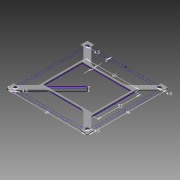
# Autodesk Inventor part: BattHolder
Saved by Autodesk Inventor 2014 SP1 (Build 180222100, 222)
## iProperties
Created: 2015-03-30
Part Number: BattHolder
Material: Generic
Document SubType Name: Modeling
Designer: Erin
Density: 1 g/cm^3
Appearance: Default
Author: Erin
Autodesk Inventor part; units mm, degrees
note: some values were not read from the file. Chosen so that the rebuilt part matches the saved one: sketch regions of "Extrusion2".
ref_plane "YZ Plane" through (0, 0, 0) normal (1, 0, 0) x (0, 1, 0)
ref_plane "XZ Plane" through (0, 0, 0) normal (0, 1, 0) x (-1, 0, 0)
ref_plane "XY Plane" through (0, 0, 0) normal (0, 0, 1) x (1, 0, 0)
sketch "Sketch1" plane through (0, 0, 0) normal (0, 0, 1) x (1, 0, 0)
  line L0 (-48, 48) -> (48, 48) construction
  line L1 (48, 48) -> (48, -48) construction
  line L2 (48, -48) -> (-48, -48) construction
  line L3 (-48, -48) -> (-48, 48) construction
  circle A0 centre (-45, 45) radius 2.25
  circle A1 centre (45, 45) radius 2.25
  line L4 (45, 45) -> (-45, 45) construction
  line L5 (-45, 45) -> (-45, -45) construction
  line L6 (-45, -45) -> (45, -45) construction
  line L7 (45, -45) -> (45, 45) construction
  circle A2 centre (45, -45) radius 2.25
  circle A3 centre (-45, -45) radius 2.25
  line L8 (-50.5, -50.5) -> (-42, -50.5)
  line L9 (-42, -50.5) -> (-42, -42)
  line L10 (-42, -42) -> (-50.5, -42)
  line L11 (-50.5, -42) -> (-50.5, -50.5)
  line L12 (0, 0) -> (-48, -48) construction
  line L13 (-33, 26.5) -> (33, 26.5)
  line L14 (33, 26.5) -> (33, -26.5)
  line L15 (33, -26.5) -> (-33, -26.5)
  line L16 (-33, -26.5) -> (-33, 26.5)
  line L17 (-2.4749, 2.4749) -> (2.4749, -2.4749)
  line L18 (2.4749, -2.4749) -> (-42.5251, -47.4749)
  line L19 (-42.5251, -47.4749) -> (-47.4749, -42.5251)
  line L20 (-47.4749, -42.5251) -> (-2.4749, 2.4749)
  line L21 (0, 0) -> (-45, -45) construction
  line L22 (31, 24.5) -> (-31, 24.5)
  line L23 (-31, 24.5) -> (-31, -24.5)
  line L24 (-31, -24.5) -> (31, -24.5)
  line L25 (31, -24.5) -> (31, 24.5)
  point P0 (0, 48)
  point P1 (48, 0)
  point P2 (33, 0)
  point P3 (0, 26.5)
  dimension "d0" = 96
  dimension "d1" = 96
  dimension "d2" = 4.5
  dimension "d3" = 4.5
  dimension "d4" = 3
  dimension "d5" = 4.5
  dimension "d6" = 4.5
  dimension "d9" = 3
  dimension "d10" = 3
  dimension "d11" = 66
  dimension "d12" = 53
  dimension "d13" = 7
  dimension "d14" = 0
  dimension "d23" = 5.5
  dimension "d24" = 5.5
  dimension "d25" = 2
  constraints: 52 end point, 12 parallel, 6 midpoint, 6 perpendicular, 4 centre point, 4 coincident, 3 horizontal, 2 horizontal alignment, 2 vertical alignment, 1 collinear, 6 other
  measures "d0" distance of L1.end L2.end
  measures "d1" distance of L0.end L1.end
  measures "d2" diameter of A0
  measures "d3" diameter of A1
  measures "d4" distance between parallel lines of L4 L0
  measures "d5" diameter of A2
  measures "d6" diameter of A3
  measures "d9" distance from line of A3.centre L10
  measures "d10" distance from line of A3.centre L9
  measures "d11" distance of L13.start L13.end
  measures "d12" distance of L13.end L14.end
  measures "d13" distance of L17.start L17.end
  measures "d14" distance from line of L5.end L19
  measures "d23" distance from line of L11 A3.centre
  measures "d24" distance from line of A3.centre L8
  measures "d25" distance between parallel lines of L22 L13
extrude "Extrusion1" add sketch "Sketch1" along normal blind 1.5 contours L20 L24 L18 L15 | L15 L16 L13 L14 L18 L24 L25 L22 L23 L20 | L24 L23 L22 L25 L18 L17 L20 | L20 L17 L18 L24
extrude "Extrusion2" add sketch "Sketch1" along normal blind 1.5 contours A3 L19 | A3 L19 L20 L10 L9 L18 | A3 L19 L18 L9 L8 L11 L10 L20 | L20 L15 L18 L9 L10 | L20 L24 L18 L15 | L20 L17 L18 L24 picked at (-45.2318, -44.2867)
extrude "Extrusion3" cut sketch "Sketch1" along normal blind 10 contours A3 L19 | L19 A3
mirror "Mirror1" about plane through (0, 0, 0) normal (1, 0, 0) of "Extrusion2", "Extrusion3"
mirror "Mirror2" about plane through (0, 0, 0) normal (0, 1, 0) of "Extrusion2", "Extrusion3", "Mirror1"
extrude "Extrusion4" cut sketch "Sketch1" along normal blind 10 contours L24 L23 L22 L25 L18 L17 L20 | L20 L17 L18 L24
fillet "Fillet3" radius 3 4 edges at (31.4497, -26.5, 0.75) (31.4497, 26.5, 0.75) (-31.4497, 26.5, 0.75) (-31.4497, -26.5, 0.75)
fillet "Fillet4" radius 10 4 edges at (-21.5503, -26.5, 0.75) (21.5503, -26.5, 0.75) (21.5503, 26.5, 0.75) (-21.5503, 26.5, 0.75)
body "Solid1"
